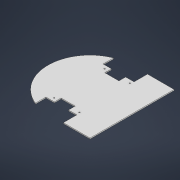
# Autodesk Inventor part: top
Saved by Autodesk Inventor 2022 (Build 260153000, 153)
## iProperties
Created: 2021-10-12
Part Number: top
Material: 一般
Document SubType Name: Modeling
Designer: shiok
Density: 1 g/cm^3
Appearance: 既定
Author: shiok
Autodesk Inventor part; units mm, degrees
ref_plane "YZ Plane" through (0, 0, 0) normal (1, 0, 0) x (0, 1, 0)
ref_plane "XZ Plane" through (0, 0, 0) normal (0, 1, 0) x (-1, 0, 0)
ref_plane "XY Plane" through (0, 0, 0) normal (0, 0, 1) x (1, 0, 0)
sketch "スケッチ1" plane through (0, 0, 0) normal (0, 1, 0) x (-1, 0, 0)
  line L0 (62.5, 0) -> (-62.5, 0)
  line L1 (-10.5, -42.5) -> (-10.5, -32.5)
  line L2 (-10.5, -32.5) -> (10.5, -32.5)
  line L3 (10.5, -32.5) -> (10.5, -42.5)
  line L4 (0, -32.5) -> (0, -42.5)
  line L5 (0, 62.5) -> (0, -62.5)
  line L6 (-10.5, 42.5) -> (-10.5, 32.5)
  line L7 (-10.5, 32.5) -> (10.5, 32.5)
  line L8 (10.5, 32.5) -> (10.5, 42.5)
  line L9 (23, -42.5) -> (10.5, -42.5)
  line L10 (-10.5, -42.5) -> (-23, -42.5)
  line L11 (23, 58.1141) -> (23, 42.5)
  line L12 (23, -42.5) -> (23, -58.1141)
  line L13 (-23, 58.1141) -> (-23, 42.5)
  line L14 (-23, -42.5) -> (-23, -58.1141)
  line L15 (23, 42.5) -> (10.5, 42.5)
  line L16 (-10.5, 42.5) -> (-23, 42.5)
  arc A0 (23, -58.1141) -> (23, 58.1141) centre (0, 0) ccw
  arc A1 (23, 58.1141) -> (23, -58.1141) centre (0, 0) ccw construction
  line L17 (-23, 62.5) -> (-23, 42.5)
  line L18 (-23, -42.5) -> (-23, -62.5)
  line L19 (-23, 62.5) -> (-62.5, 62.5)
  line L20 (-62.5, 62.5) -> (-62.5, -62.5)
  line L21 (-62.5, -62.5) -> (-23, -62.5)
  point P0 (15.75, -37.5)
  point P1 (-21.75, -37.5)
  point P2 (15.75, 37.5)
  point P3 (-21.75, 37.5)
  dimension "d1" = 37.5
  dimension "d2" = 21.75
  dimension "d4" = 37.5
  dimension "d8" = 21
  dimension "d9" = 10
  dimension "d25" = 65
  dimension "d27" = 23
  dimension "d30" = 62.5
  dimension "d31" = 23
  constraints: 44 end point, 10 point on circle, 8 symmetric about line, 7 perpendicular, 5 parallel, 4 midpoint, 3 point on line, 3 tangent, 3 vertical, 2 centre point, 2 collinear, 2 horizontal, 1 coincident, 1 horizontal alignment
  measures "d1" distance of point (-21.75, -37.5) point (15.75, -37.5)
  measures "d2" horizontal distance of point (0, 0) point (-21.75, -37.5)
  measures "d4" vertical distance of point (0, 0) point (-21.75, -37.5)
  measures "d8" distance between parallel lines of L1 L3
  measures "d9" distance of L3.end L2.end
  measures "d25" distance between parallel lines of L7 L2
  measures "d27" distance from line of L12 point (0, 0)
  measures "d30" radius of A0
  measures "d31" distance from line of point (0, 0) L14
extrude "押し出し1" add sketch "スケッチ1" along normal blind 1.4
sketch "スケッチ2" plane through (0, 1.4, 0) normal (0, 1, 0) x (1, 0, 0)
  line L0 (62.5, 0) -> (-62.5, 0)
  point P0 (0, 0)
  point P1 (0, 0)
  point P2 (-15.75, 37.5)
  point P3 (21.75, 37.5)
  point P4 (0, 0)
  point P5 (21.75, -37.5)
  point P6 (-15.75, -37.5)
  dimension "d14" = 37.5
  dimension "d15" = 21.75
  dimension "d16" = 37.5
  constraints: 2 end point, 2 midpoint, 2 symmetric about line, 1 horizontal
  measures "d14" distance of point (21.75, 37.5) point (-15.75, 37.5)
  measures "d15" horizontal distance of point (0, 0) point (21.75, 37.5)
  measures "d16" vertical distance of point (0, 0) point (21.75, 37.5)
hole "穴1" at (21.75, 1.4, -37.5) at (-15.75, 1.4, -37.5) at (-15.75, 1.4, 37.5) at (21.75, 1.4, 37.5) direction (0, -1, 0) diameter 1.778 end through all clearance for "Flat Head Machine Screw (82)" size "#0" standard "Ansi Unified Screw Threads"
